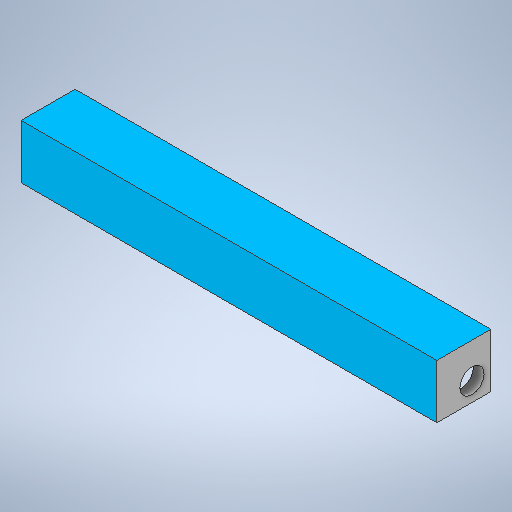
# Autodesk Inventor part: Legs
Saved by Autodesk Inventor 2025.1 (Build 291241020, 241B)
## iProperties
Created: 2024-10-28
Part Number: Legs
Material: Generic
Document SubType Name: Modeling
Designer: nitve
Density: 1 g/cm^3
Appearance: Default
Author: nitve
Autodesk Inventor part; units mm, degrees
ref_plane "YZ Plane" through (0, 0, 0) normal (1, 0, 0) x (0, 1, 0)
ref_plane "XZ Plane" through (0, 0, 0) normal (0, 1, 0) x (-1, 0, 0)
ref_plane "XY Plane" through (0, 0, 0) normal (0, 0, 1) x (1, 0, 0)
sketch "Sketch1" plane through (0, 0, 0) normal (0, 1, 0) x (-1, 0, 0)
  line L0 (0, 0) -> (77, 0)
  line L1 (77, 0) -> (77, -10)
  line L2 (77, -10) -> (0, -10)
  line L3 (0, -10) -> (0, 0)
  line L4 (77, 0) -> (0, 0)
  line L5 (0, 0) -> (0, -2)
  line L6 (0, -2) -> (77, -2)
  line L7 (77, -2) -> (77, 0)
  point P0 (77, -2)
  point P1 (77, -5)
  dimension "d1" = 10
  dimension "d3" = 2
  dimension "d19" = 77
  constraints: 16 end point, 4 parallel, 2 horizontal, 2 perpendicular, 1 midpoint, 1 point on line
  measures "d1" distance of L2.end L0.start
  measures "d3" distance of L0.start L5.end
  measures "d19" distance from line of L3 point (77, -5)
extrude "Extrusion1" add sketch "Sketch1" along normal blind 2 contours L6 L1 L2 L3
extrude "Extrusion2" add sketch "Sketch1" along normal blind 10 contours L0 L1 L6 L3
sketch "Sketch2" plane through (0, 0, -10) normal (1, 0, 0) x (0, 0, -1)
  line L0 (-10, 0) -> (0, 0) projected
  line L1 (-10, 0) -> (0, 0)
  line L2 (0, 0) -> (0, 10)
  line L3 (0, 10) -> (-10, 10)
  line L4 (-10, 10) -> (-10, 0)
  dimension "d8" = 10
  dimension "d9" = 10
  constraints: 8 end point, 2 parallel, 1 horizontal, 1 perpendicular
  measures "d8" distance of L2.end L3.end
  measures "d9" distance of L1.end L2.end
extrude "Extrusion3" add sketch "Sketch2" against normal blind 2
sketch "Sketch3" plane through (-77, 0, -10) normal (-1, 0, 0) x (0, 0, 1)
  line L0 (0, 0) -> (0, 10) projected
  line L1 (10, 10) -> (0, 10) projected
  line L2 (0, 0) -> (10, 0)
  line L3 (10, 0) -> (10, 10)
  line L4 (10, 10) -> (0, 10)
  line L5 (0, 10) -> (0, 0)
  point P0 (10, 0)
  constraints: 8 end point, 2 parallel, 1 horizontal, 1 perpendicular
extrude "Extrusion4" add sketch "Sketch3" against normal blind 2
sketch "Sketch5" plane through (0, 0, 0) normal (1, 0, 0) x (0, 0, -1)
  line L0 (0, 10) -> (10, 10) projected
  line L1 (10, 0) -> (10, 10) projected
  point P0 (0, 0)
  point P1 (6.5, 6.5)
  dimension "d23" = 3.5
  dimension "d24" = 3.5
  measures "d23" distance from line of L0 point (6.5, 6.5)
  measures "d24" distance from line of L1 point (6.5, 6.5)
hole "Hole1" at (0, 6.5, -6.5) direction (-1, 0, 0) diameter 4.5 end through all clearance for "Flat Head Machine Screw" size "M4" standard "Ansi Metric M Profile"
body "Solid1"
